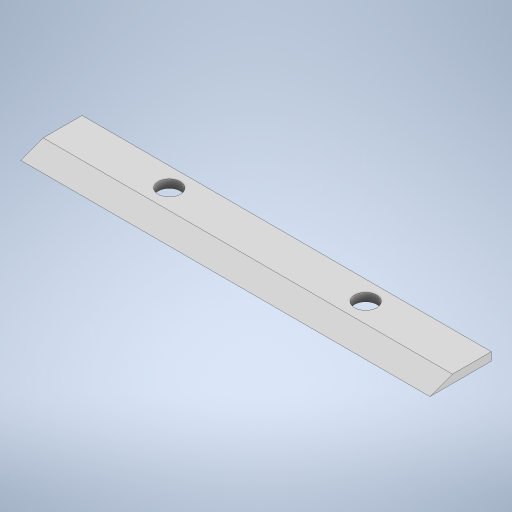
# Autodesk Inventor part: Blade
Saved by Autodesk Inventor 2024 (Build 280153000, 153)
## iProperties
Created: 2024-01-20
Part Number: Blade
Material: Generic
Document SubType Name: Modeling
Designer: kdcao
Density: 1 g/cm^3
Appearance: Default
Author: kdcao
Autodesk Inventor part; units mm, degrees
ref_plane "YZ Plane" through (0, 0, 0) normal (1, 0, 0) x (0, 1, 0)
ref_plane "XZ Plane" through (0, 0, 0) normal (0, 1, 0) x (-1, 0, 0)
sketch "Sketch1" plane through (0, 0, 0) normal (0, 1, 0) x (-1, 0, 0)
  line L0 (0, 0) -> (100, 0)
  line L1 (100, 0) -> (100, -15)
  line L2 (100, -15) -> (0, -15)
  line L3 (0, -15) -> (0, 0)
  dimension "d0" = 100
  dimension "d1" = 15
  constraints: 8 end point, 2 parallel, 1 horizontal, 1 perpendicular
  measures "d0" distance of L1.end L2.end
  measures "d1" distance of L0.end L1.end
extrude "Extrusion1" add sketch "Sketch1" along normal blind 2
sketch "Sketch2" plane through (0, 0, 0) normal (1, 0, 0) x (0, 0, -1)
  line L0 (0, 0) -> (0, 2) projected
  line L1 (0, 0) -> (5.495, 2)
  line L2 (5.495, 2) -> (5.495, 0)
  line L3 (5.495, 0) -> (0, 0)
  line L4 (0, 2) -> (15, 2) projected
  dimension "d4" = 20
  constraints: 6 end point, 1 perpendicular, 1 point on line, 1 vertical
  measures "d4" angle of L3 L1
extrude "Extrusion2" cut sketch "Sketch2" against normal through all contours L0 L4 L1
sketch "Sketch3" plane through (0, 2, 0) normal (0, 1, 0) x (1, 0, 0)
  line L0 (-100, 15) -> (-100, 5.495) projected
  point P0 (0, 0)
  point P1 (-74, 10.3)
  point P2 (-100, 10.2475)
  dimension "d14" = 26
  dimension "d15" = 4.7
  constraints: 1 midpoint
  measures "d14" horizontal distance of point (-100, 10.247) point (-74, 10.3)
  measures "d15" vertical distance of L0.start point (-74, 10.3)
hole "Hole1" at (-74, 2, -10.3) direction (0, -1, 0) diameter 5.4 depth 5.83
ref_plane "Work Plane1" through (-50, 0, -15) normal (1, 0, 0) x (0, 0, -1)
mirror "Mirror1" about plane through (-50, 0, -15) normal (1, 0, 0) of "Hole1"
body "Solid1"
